Autodesk Inventor part; units mm, degrees
(part 3 of 13)
  arc A798 (17.121, 51.219) -> (17.121, 51.345) centre (17.121, 51.282) ccw
  line L797 (17.121, 51.345) -> (3.5797, 51.345)
  arc A799 (3.5797, 51.345) -> (3.5797, 51.219) centre (3.5797, 51.282) ccw
  line L798 (1.0789, 51.345) -> (1.2725, 51.345)
  arc A800 (1.2725, 51.345) -> (1.2725, 51.471) centre (1.2725, 51.408) ccw
  line L799 (1.2725, 51.471) -> (1.0789, 51.471)
  arc A801 (1.0789, 51.471) -> (1.0789, 51.345) centre (1.0789, 51.408) ccw
  line L800 (2.337, 51.345) -> (2.4628, 51.345)
  arc A802 (2.4628, 51.345) -> (2.4628, 51.471) centre (2.4628, 51.408) ccw
  line L801 (2.4628, 51.471) -> (2.337, 51.471)
  arc A803 (2.337, 51.471) -> (2.337, 51.345) centre (2.337, 51.408) ccw
  line L802 (3.5275, 51.345) -> (17.121, 51.345)
  arc A804 (17.121, 51.345) -> (17.121, 51.471) centre (17.121, 51.408) ccw
  line L803 (17.121, 51.471) -> (3.5275, 51.471)
  arc A805 (3.5275, 51.471) -> (3.5275, 51.345) centre (3.5275, 51.408) ccw
  line L804 (1.0789, 51.471) -> (1.3247, 51.471)
  arc A806 (1.3247, 51.471) -> (1.3247, 51.597) centre (1.3247, 51.534) ccw
  line L805 (1.3247, 51.597) -> (1.0789, 51.597)
  arc A807 (1.0789, 51.597) -> (1.0789, 51.471) centre (1.0789, 51.534) ccw
  line L806 (2.337, 51.471) -> (2.4628, 51.471)
  arc A808 (2.4628, 51.471) -> (2.4628, 51.597) centre (2.4628, 51.534) ccw
  line L807 (2.4628, 51.597) -> (2.337, 51.597)
  arc A809 (2.337, 51.597) -> (2.337, 51.471) centre (2.337, 51.534) ccw
  line L808 (3.4753, 51.471) -> (17.121, 51.471)
  arc A810 (17.121, 51.471) -> (17.121, 51.597) centre (17.121, 51.534) ccw
  line L809 (17.121, 51.597) -> (3.4753, 51.597)
  arc A811 (3.4753, 51.597) -> (3.4753, 51.471) centre (3.4753, 51.534) ccw
  line L810 (1.0789, 51.597) -> (1.389, 51.597)
  arc A812 (1.389, 51.597) -> (1.389, 51.723) centre (1.389, 51.66) ccw
  line L811 (1.389, 51.723) -> (1.0789, 51.723)
  arc A813 (1.0789, 51.723) -> (1.0789, 51.597) centre (1.0789, 51.66) ccw
  line L812 (2.337, 51.597) -> (2.4628, 51.597)
  arc A814 (2.4628, 51.597) -> (2.4628, 51.723) centre (2.4628, 51.66) ccw
  line L813 (2.4628, 51.723) -> (2.337, 51.723)
  arc A815 (2.337, 51.723) -> (2.337, 51.597) centre (2.337, 51.66) ccw
  line L814 (3.4109, 51.597) -> (17.121, 51.597)
  arc A816 (17.121, 51.597) -> (17.121, 51.723) centre (17.121, 51.66) ccw
  line L815 (17.121, 51.723) -> (3.4109, 51.723)
  arc A817 (3.4109, 51.723) -> (3.4109, 51.597) centre (3.4109, 51.66) ccw
  line L816 (1.0789, 51.723) -> (1.515, 51.723)
  arc A818 (1.515, 51.723) -> (1.515, 51.849) centre (1.515, 51.786) ccw
  line L817 (1.515, 51.849) -> (1.0789, 51.849)
  arc A819 (1.0789, 51.849) -> (1.0789, 51.723) centre (1.0789, 51.786) ccw
  line L818 (2.337, 51.723) -> (2.4628, 51.723)
  arc A820 (2.4628, 51.723) -> (2.4628, 51.849) centre (2.4628, 51.786) ccw
  line L819 (2.4628, 51.849) -> (2.337, 51.849)
  arc A821 (2.337, 51.849) -> (2.337, 51.723) centre (2.337, 51.786) ccw
  line L820 (3.2849, 51.723) -> (17.121, 51.723)
  arc A822 (17.121, 51.723) -> (17.121, 51.849) centre (17.121, 51.786) ccw
  line L821 (17.121, 51.849) -> (3.2849, 51.849)
  arc A823 (3.2849, 51.849) -> (3.2849, 51.723) centre (3.2849, 51.786) ccw
  line L822 (1.0789, 51.849) -> (1.641, 51.849)
  arc A824 (1.641, 51.849) -> (1.641, 51.975) centre (1.641, 51.912) ccw
  line L823 (1.641, 51.975) -> (1.0789, 51.975)
  arc A825 (1.0789, 51.975) -> (1.0789, 51.849) centre (1.0789, 51.912) ccw
  line L824 (2.337, 51.849) -> (2.4628, 51.849)
  arc A826 (2.4628, 51.849) -> (2.4628, 51.975) centre (2.4628, 51.912) ccw
  line L825 (2.4628, 51.975) -> (2.337, 51.975)
  arc A827 (2.337, 51.975) -> (2.337, 51.849) centre (2.337, 51.912) ccw
  line L826 (3.1589, 51.849) -> (17.121, 51.849)
  arc A828 (17.121, 51.849) -> (17.121, 51.975) centre (17.121, 51.912) ccw
  line L827 (17.121, 51.975) -> (3.1589, 51.975)
  arc A829 (3.1589, 51.975) -> (3.1589, 51.849) centre (3.1589, 51.912) ccw
  line L828 (1.0789, 51.975) -> (1.8468, 51.975)
  arc A830 (1.8468, 51.975) -> (1.8468, 52.101) centre (1.8468, 52.038) ccw
  line L829 (1.8468, 52.101) -> (1.0789, 52.101)
  arc A831 (1.0789, 52.101) -> (1.0789, 51.975) centre (1.0789, 52.038) ccw
  line L830 (2.337, 51.975) -> (2.4628, 51.975)
  arc A832 (2.4628, 51.975) -> (2.4628, 52.101) centre (2.4628, 52.038) ccw
  line L831 (2.4628, 52.101) -> (2.337, 52.101)
  arc A833 (2.337, 52.101) -> (2.337, 51.975) centre (2.337, 52.038) ccw
  line L832 (2.9532, 51.975) -> (17.121, 51.975)
  arc A834 (17.121, 51.975) -> (17.121, 52.101) centre (17.121, 52.038) ccw
  line L833 (17.121, 52.101) -> (2.9532, 52.101)
  arc A835 (2.9532, 52.101) -> (2.9532, 51.975) centre (2.9532, 52.038) ccw
  line L834 (1.0789, 52.101) -> (2.1509, 52.101)
  arc A836 (2.1509, 52.101) -> (2.1509, 52.227) centre (2.1509, 52.164) ccw
  line L835 (2.1509, 52.227) -> (1.0789, 52.227)
  arc A837 (1.0789, 52.227) -> (1.0789, 52.101) centre (1.0789, 52.164) ccw
  line L836 (2.337, 52.101) -> (2.4628, 52.101)
  arc A838 (2.4628, 52.101) -> (2.4628, 52.227) centre (2.4628, 52.164) ccw
  line L837 (2.4628, 52.227) -> (2.337, 52.227)
  arc A839 (2.337, 52.227) -> (2.337, 52.101) centre (2.337, 52.164) ccw
  line L838 (2.6491, 52.101) -> (17.121, 52.101)
  arc A840 (17.121, 52.101) -> (17.121, 52.227) centre (17.121, 52.164) ccw
  line L839 (17.121, 52.227) -> (2.6491, 52.227)
  arc A841 (2.6491, 52.227) -> (2.6491, 52.101) centre (2.6491, 52.164) ccw
  line L840 (1.0789, 52.227) -> (17.121, 52.227)
  arc A842 (17.121, 52.227) -> (17.121, 52.353) centre (17.121, 52.29) ccw
  line L841 (17.121, 52.353) -> (1.0789, 52.353)
  arc A843 (1.0789, 52.353) -> (1.0789, 52.227) centre (1.0789, 52.29) ccw
  line L842 (1.0789, 52.353) -> (17.121, 52.353)
  arc A844 (17.121, 52.353) -> (17.121, 52.479) centre (17.121, 52.416) ccw
  line L843 (17.121, 52.479) -> (1.0789, 52.479)
  arc A845 (1.0789, 52.479) -> (1.0789, 52.353) centre (1.0789, 52.416) ccw
  line L844 (1.0789, 52.479) -> (17.121, 52.479)
  arc A846 (17.121, 52.479) -> (17.121, 52.605) centre (17.121, 52.542) ccw
  line L845 (17.121, 52.605) -> (1.0789, 52.605)
  arc A847 (1.0789, 52.605) -> (1.0789, 52.479) centre (1.0789, 52.542) ccw
  line L846 (1.0789, 52.605) -> (17.121, 52.605)
  arc A848 (17.121, 52.605) -> (17.121, 52.731) centre (17.121, 52.668) ccw
  line L847 (17.121, 52.731) -> (1.0789, 52.731)
  arc A849 (1.0789, 52.731) -> (1.0789, 52.605) centre (1.0789, 52.668) ccw
  line L848 (1.0789, 52.731) -> (17.121, 52.731)
  arc A850 (17.121, 52.731) -> (17.121, 52.857) centre (17.121, 52.794) ccw
  line L849 (17.121, 52.857) -> (1.0789, 52.857)
  arc A851 (1.0789, 52.857) -> (1.0789, 52.731) centre (1.0789, 52.794) ccw
  line L850 (1.0789, 52.857) -> (17.121, 52.857)
  arc A852 (17.121, 52.857) -> (17.121, 52.983) centre (17.121, 52.92) ccw
  line L851 (17.121, 52.983) -> (1.0789, 52.983)
  arc A853 (1.0789, 52.983) -> (1.0789, 52.857) centre (1.0789, 52.92) ccw
  line L852 (1.0789, 52.983) -> (17.121, 52.983)
  arc A854 (17.121, 52.983) -> (17.121, 53.109) centre (17.121, 53.046) ccw
  line L853 (17.121, 53.109) -> (1.0789, 53.109)
  arc A855 (1.0789, 53.109) -> (1.0789, 52.983) centre (1.0789, 53.046) ccw
  line L854 (1.0789, 53.109) -> (17.121, 53.109)
  arc A856 (17.121, 53.109) -> (17.121, 53.235) centre (17.121, 53.172) ccw
  line L855 (17.121, 53.235) -> (1.0789, 53.235)
  arc A857 (1.0789, 53.235) -> (1.0789, 53.109) centre (1.0789, 53.172) ccw
  line L856 (1.0789, 53.235) -> (17.121, 53.235)
  arc A858 (17.121, 53.235) -> (17.121, 53.361) centre (17.121, 53.298) ccw
  line L857 (17.121, 53.361) -> (1.0789, 53.361)
  arc A859 (1.0789, 53.361) -> (1.0789, 53.235) centre (1.0789, 53.298) ccw
  line L858 (1.0789, 53.361) -> (1.9622, 53.361)
  arc A860 (1.9622, 53.361) -> (1.9622, 53.487) centre (1.9622, 53.424) ccw
  line L859 (1.9622, 53.487) -> (1.0789, 53.487)
  arc A861 (1.0789, 53.487) -> (1.0789, 53.361) centre (1.0789, 53.424) ccw
  line L860 (2.8376, 53.361) -> (17.121, 53.361)
  arc A862 (17.121, 53.361) -> (17.121, 53.487) centre (17.121, 53.424) ccw
  line L861 (17.121, 53.487) -> (2.8376, 53.487)
  arc A863 (2.8376, 53.487) -> (2.8376, 53.361) centre (2.8376, 53.424) ccw
  line L862 (1.0789, 53.487) -> (1.7225, 53.487)
  arc A864 (1.7225, 53.487) -> (1.7225, 53.613) centre (1.7225, 53.55) ccw
  line L863 (1.7225, 53.613) -> (1.0789, 53.613)
  arc A865 (1.0789, 53.613) -> (1.0789, 53.487) centre (1.0789, 53.55) ccw
  line L864 (3.0774, 53.487) -> (17.121, 53.487)
  arc A866 (17.121, 53.487) -> (17.121, 53.613) centre (17.121, 53.55) ccw
  line L865 (17.121, 53.613) -> (3.0774, 53.613)
  arc A867 (3.0774, 53.613) -> (3.0774, 53.487) centre (3.0774, 53.55) ccw
  line L866 (1.0789, 53.613) -> (1.5965, 53.613)
  arc A868 (1.5965, 53.613) -> (1.5965, 53.739) centre (1.5965, 53.676) ccw
  line L867 (1.5965, 53.739) -> (1.0789, 53.739)
  arc A869 (1.0789, 53.739) -> (1.0789, 53.613) centre (1.0789, 53.676) ccw
  line L868 (3.2034, 53.613) -> (7.2516, 53.613)
  arc A870 (7.2516, 53.613) -> (7.2516, 53.739) centre (7.2516, 53.676) ccw
  line L869 (7.2516, 53.739) -> (3.2034, 53.739)
  arc A871 (3.2034, 53.739) -> (3.2034, 53.613) centre (3.2034, 53.676) ccw
  line L870 (8.1482, 53.613) -> (17.121, 53.613)
  arc A872 (17.121, 53.613) -> (17.121, 53.739) centre (17.121, 53.676) ccw
  line L871 (17.121, 53.739) -> (8.1482, 53.739)
  arc A873 (8.1482, 53.739) -> (8.1482, 53.613) centre (8.1482, 53.676) ccw
  line L872 (1.0789, 53.739) -> (1.4705, 53.739)
  arc A874 (1.4705, 53.739) -> (1.4705, 53.865) centre (1.4705, 53.802) ccw
  line L873 (1.4705, 53.865) -> (1.0789, 53.865)
  arc A875 (1.0789, 53.865) -> (1.0789, 53.739) centre (1.0789, 53.802) ccw
  line L874 (3.3294, 53.739) -> (6.9684, 53.739)
  arc A876 (6.9684, 53.739) -> (6.9684, 53.865) centre (6.9684, 53.802) ccw
  line L875 (6.9684, 53.865) -> (3.3294, 53.865)
  arc A877 (3.3294, 53.865) -> (3.3294, 53.739) centre (3.3294, 53.802) ccw
  line L876 (8.4315, 53.739) -> (17.121, 53.739)
  arc A878 (17.121, 53.739) -> (17.121, 53.865) centre (17.121, 53.802) ccw
  line L877 (17.121, 53.865) -> (8.4315, 53.865)
  arc A879 (8.4315, 53.865) -> (8.4315, 53.739) centre (8.4315, 53.802) ccw
  line L878 (1.0789, 53.865) -> (1.4088, 53.865)
  arc A880 (1.4088, 53.865) -> (1.4088, 53.991) centre (1.4088, 53.928) ccw
  line L879 (1.4088, 53.991) -> (1.0789, 53.991)
  arc A881 (1.0789, 53.991) -> (1.0789, 53.865) centre (1.0789, 53.928) ccw
  line L880 (3.391, 53.865) -> (6.8424, 53.865)
  arc A882 (6.8424, 53.865) -> (6.8424, 53.991) centre (6.8424, 53.928) ccw
  line L881 (6.8424, 53.991) -> (3.391, 53.991)
  arc A883 (3.391, 53.991) -> (3.391, 53.865) centre (3.391, 53.928) ccw
  line L882 (8.5575, 53.865) -> (17.121, 53.865)
  arc A884 (17.121, 53.865) -> (17.121, 53.991) centre (17.121, 53.928) ccw
  line L883 (17.121, 53.991) -> (8.5575, 53.991)
  arc A885 (8.5575, 53.991) -> (8.5575, 53.865) centre (8.5575, 53.928) ccw
  line L884 (1.0789, 53.991) -> (1.3567, 53.991)
  arc A886 (1.3567, 53.991) -> (1.3567, 54.117) centre (1.3567, 54.054) ccw
  line L885 (1.3567, 54.117) -> (1.0789, 54.117)
  arc A887 (1.0789, 54.117) -> (1.0789, 53.991) centre (1.0789, 54.054) ccw
  line L886 (3.4431, 53.991) -> (6.7164, 53.991)
  arc A888 (6.7164, 53.991) -> (6.7164, 54.117) centre (6.7164, 54.054) ccw
  line L887 (6.7164, 54.117) -> (3.4431, 54.117)
  arc A889 (3.4431, 54.117) -> (3.4431, 53.991) centre (3.4431, 54.054) ccw
  line L888 (8.6835, 53.991) -> (17.121, 53.991)
  arc A890 (17.121, 53.991) -> (17.121, 54.117) centre (17.121, 54.054) ccw
  line L889 (17.121, 54.117) -> (8.6835, 54.117)
  arc A891 (8.6835, 54.117) -> (8.6835, 53.991) centre (8.6835, 54.054) ccw
  line L890 (1.0789, 54.117) -> (1.3045, 54.117)
  arc A892 (1.3045, 54.117) -> (1.3045, 54.243) centre (1.3045, 54.18) ccw
  line L891 (1.3045, 54.243) -> (1.0789, 54.243)
  arc A893 (1.0789, 54.243) -> (1.0789, 54.117) centre (1.0789, 54.18) ccw
  line L892 (3.4953, 54.117) -> (6.6119, 54.117)
  arc A894 (6.6119, 54.117) -> (6.6119, 54.243) centre (6.6119, 54.18) ccw
  line L893 (6.6119, 54.243) -> (3.4953, 54.243)
  arc A895 (3.4953, 54.243) -> (3.4953, 54.117) centre (3.4953, 54.18) ccw
  line L894 (8.7879, 54.117) -> (17.121, 54.117)
  arc A896 (17.121, 54.117) -> (17.121, 54.243) centre (17.121, 54.18) ccw
  line L895 (17.121, 54.243) -> (8.7879, 54.243)
  arc A897 (8.7879, 54.243) -> (8.7879, 54.117) centre (8.7879, 54.18) ccw
  line L896 (1.0789, 54.243) -> (1.2846, 54.243)
  arc A898 (1.2846, 54.243) -> (1.2846, 54.369) centre (1.2846, 54.306) ccw
  line L897 (1.2846, 54.369) -> (1.0789, 54.369)
  arc A899 (1.0789, 54.369) -> (1.0789, 54.243) centre (1.0789, 54.306) ccw
  line L898 (3.5153, 54.243) -> (6.5597, 54.243)
  arc A900 (6.5597, 54.243) -> (6.5597, 54.369) centre (6.5597, 54.306) ccw
  line L899 (6.5597, 54.369) -> (3.5153, 54.369)
  arc A901 (3.5153, 54.369) -> (3.5153, 54.243) centre (3.5153, 54.306) ccw
  line L900 (8.8401, 54.243) -> (17.121, 54.243)
  arc A902 (17.121, 54.243) -> (17.121, 54.369) centre (17.121, 54.306) ccw
  line L901 (17.121, 54.369) -> (8.8401, 54.369)
  arc A903 (8.8401, 54.369) -> (8.8401, 54.243) centre (8.8401, 54.306) ccw
  line L902 (1.0789, 54.369) -> (1.2846, 54.369)
  arc A904 (1.2846, 54.369) -> (1.2846, 54.495) centre (1.2846, 54.432) ccw
  line L903 (1.2846, 54.495) -> (1.0789, 54.495)
  arc A905 (1.0789, 54.495) -> (1.0789, 54.369) centre (1.0789, 54.432) ccw
  line L904 (3.5153, 54.369) -> (6.5075, 54.369)
  arc A906 (6.5075, 54.369) -> (6.5075, 54.495) centre (6.5075, 54.432) ccw
  line L905 (6.5075, 54.495) -> (3.5153, 54.495)
  arc A907 (3.5153, 54.495) -> (3.5153, 54.369) centre (3.5153, 54.432) ccw
  line L906 (8.8923, 54.369) -> (17.121, 54.369)
  arc A908 (17.121, 54.369) -> (17.121, 54.495) centre (17.121, 54.432) ccw
  line L907 (17.121, 54.495) -> (8.8923, 54.495)
  arc A909 (8.8923, 54.495) -> (8.8923, 54.369) centre (8.8923, 54.432) ccw
  line L908 (1.0789, 54.495) -> (1.2846, 54.495)
  arc A910 (1.2846, 54.495) -> (1.2846, 54.621) centre (1.2846, 54.558) ccw
  line L909 (1.2846, 54.621) -> (1.0789, 54.621)
  arc A911 (1.0789, 54.621) -> (1.0789, 54.495) centre (1.0789, 54.558) ccw
  line L910 (3.5153, 54.495) -> (6.4553, 54.495)
  arc A912 (6.4553, 54.495) -> (6.4553, 54.621) centre (6.4553, 54.558) ccw
  line L911 (6.4553, 54.621) -> (3.5153, 54.621)
  arc A913 (3.5153, 54.621) -> (3.5153, 54.495) centre (3.5153, 54.558) ccw
  line L912 (8.9445, 54.495) -> (17.121, 54.495)
  arc A914 (17.121, 54.495) -> (17.121, 54.621) centre (17.121, 54.558) ccw
  line L913 (17.121, 54.621) -> (8.9445, 54.621)
  arc A915 (8.9445, 54.621) -> (8.9445, 54.495) centre (8.9445, 54.558) ccw
  line L914 (1.0789, 54.621) -> (1.2897, 54.621)
  arc A916 (1.2897, 54.621) -> (1.2897, 54.747) centre (1.2897, 54.684) ccw
  line L915 (1.2897, 54.747) -> (1.0789, 54.747)
  arc A917 (1.0789, 54.747) -> (1.0789, 54.621) centre (1.0789, 54.684) ccw
  line L916 (3.5103, 54.621) -> (6.4346, 54.621)
  arc A918 (6.4346, 54.621) -> (6.4346, 54.747) centre (6.4346, 54.684) ccw
  line L917 (6.4346, 54.747) -> (3.5103, 54.747)
  arc A919 (3.5103, 54.747) -> (3.5103, 54.621) centre (3.5103, 54.684) ccw
  line L918 (8.9653, 54.621) -> (17.121, 54.621)
  arc A920 (17.121, 54.621) -> (17.121, 54.747) centre (17.121, 54.684) ccw
  line L919 (17.121, 54.747) -> (8.9653, 54.747)
  arc A921 (8.9653, 54.747) -> (8.9653, 54.621) centre (8.9653, 54.684) ccw
  line L920 (1.0789, 54.747) -> (1.3419, 54.747)
  arc A922 (1.3419, 54.747) -> (1.3419, 54.873) centre (1.3419, 54.81) ccw
  line L921 (1.3419, 54.873) -> (1.0789, 54.873)
  arc A923 (1.0789, 54.873) -> (1.0789, 54.747) centre (1.0789, 54.81) ccw
  line L922 (3.4581, 54.747) -> (6.4346, 54.747)
  arc A924 (6.4346, 54.747) -> (6.4346, 54.873) centre (6.4346, 54.81) ccw
  line L923 (6.4346, 54.873) -> (3.4581, 54.873)
  arc A925 (3.4581, 54.873) -> (3.4581, 54.747) centre (3.4581, 54.81) ccw
  line L924 (8.9653, 54.747) -> (17.121, 54.747)
  arc A926 (17.121, 54.747) -> (17.121, 54.873) centre (17.121, 54.81) ccw
  line L925 (17.121, 54.873) -> (8.9653, 54.873)
  arc A927 (8.9653, 54.873) -> (8.9653, 54.747) centre (8.9653, 54.81) ccw
  line L926 (1.0789, 54.873) -> (1.3941, 54.873)
  arc A928 (1.3941, 54.873) -> (1.3941, 54.999) centre (1.3941, 54.936) ccw
  line L927 (1.3941, 54.999) -> (1.0789, 54.999)
  arc A929 (1.0789, 54.999) -> (1.0789, 54.873) centre (1.0789, 54.936) ccw
  line L928 (3.4059, 54.873) -> (6.4346, 54.873)
  arc A930 (6.4346, 54.873) -> (6.4346, 54.999) centre (6.4346, 54.936) ccw
  line L929 (6.4346, 54.999) -> (3.4059, 54.999)
  arc A931 (3.4059, 54.999) -> (3.4059, 54.873) centre (3.4059, 54.936) ccw
  line L930 (8.9653, 54.873) -> (17.121, 54.873)
  arc A932 (17.121, 54.873) -> (17.121, 54.999) centre (17.121, 54.936) ccw
  line L931 (17.121, 54.999) -> (8.9653, 54.999)
  arc A933 (8.9653, 54.999) -> (8.9653, 54.873) centre (8.9653, 54.936) ccw
  line L932 (1.0789, 54.999) -> (1.4462, 54.999)
  arc A934 (1.4462, 54.999) -> (1.4462, 55.125) centre (1.4462, 55.062) ccw
  line L933 (1.4462, 55.125) -> (1.0789, 55.125)
  arc A935 (1.0789, 55.125) -> (1.0789, 54.999) centre (1.0789, 55.062) ccw
  line L934 (3.3538, 54.999) -> (6.4346, 54.999)
  arc A936 (6.4346, 54.999) -> (6.4346, 55.125) centre (6.4346, 55.062) ccw
  line L935 (6.4346, 55.125) -> (3.3538, 55.125)
  arc A937 (3.3538, 55.125) -> (3.3538, 54.999) centre (3.3538, 55.062) ccw
  line L936 (8.9653, 54.999) -> (17.121, 54.999)
  arc A938 (17.121, 54.999) -> (17.121, 55.125) centre (17.121, 55.062) ccw
  line L937 (17.121, 55.125) -> (8.9653, 55.125)
  arc A939 (8.9653, 55.125) -> (8.9653, 54.999) centre (8.9653, 55.062) ccw
  line L938 (1.0789, 55.125) -> (1.5606, 55.125)
  arc A940 (1.5606, 55.125) -> (1.5606, 55.251) centre (1.5606, 55.188) ccw
  line L939 (1.5606, 55.251) -> (1.0789, 55.251)
  arc A941 (1.0789, 55.251) -> (1.0789, 55.125) centre (1.0789, 55.188) ccw
  line L940 (3.2393, 55.125) -> (6.4663, 55.125)
  arc A942 (6.4663, 55.125) -> (6.4663, 55.251) centre (6.4663, 55.188) ccw
  line L941 (6.4663, 55.251) -> (3.2393, 55.251)
  arc A943 (3.2393, 55.251) -> (3.2393, 55.125) centre (3.2393, 55.188) ccw
  line L942 (8.9337, 55.125) -> (17.121, 55.125)
  arc A944 (17.121, 55.125) -> (17.121, 55.251) centre (17.121, 55.188) ccw
  line L943 (17.121, 55.251) -> (8.9337, 55.251)
  arc A945 (8.9337, 55.251) -> (8.9337, 55.125) centre (8.9337, 55.188) ccw
  line L944 (1.0789, 55.251) -> (1.6866, 55.251)
  arc A946 (1.6866, 55.251) -> (1.6866, 55.377) centre (1.6866, 55.314) ccw
  line L945 (1.6866, 55.377) -> (1.0789, 55.377)
  arc A947 (1.0789, 55.377) -> (1.0789, 55.251) centre (1.0789, 55.314) ccw
  line L946 (3.1133, 55.251) -> (6.5184, 55.251)
  arc A948 (6.5184, 55.251) -> (6.5184, 55.377) centre (6.5184, 55.314) ccw
  line L947 (6.5184, 55.377) -> (3.1133, 55.377)
  arc A949 (3.1133, 55.377) -> (3.1133, 55.251) centre (3.1133, 55.314) ccw
  line L948 (8.8816, 55.251) -> (17.121, 55.251)
  arc A950 (17.121, 55.251) -> (17.121, 55.377) centre (17.121, 55.314) ccw
  line L949 (17.121, 55.377) -> (8.8816, 55.377)
  arc A951 (8.8816, 55.377) -> (8.8816, 55.251) centre (8.8816, 55.314) ccw
  line L950 (1.0789, 55.377) -> (1.8756, 55.377)
  arc A952 (1.8756, 55.377) -> (1.8756, 55.503) centre (1.8756, 55.44) ccw
  line L951 (1.8756, 55.503) -> (1.0789, 55.503)
  arc A953 (1.0789, 55.503) -> (1.0789, 55.377) centre (1.0789, 55.44) ccw
  line L952 (2.9244, 55.377) -> (6.5706, 55.377)
  arc A954 (6.5706, 55.377) -> (6.5706, 55.503) centre (6.5706, 55.44) ccw
  line L953 (6.5706, 55.503) -> (2.9244, 55.503)
  arc A955 (2.9244, 55.503) -> (2.9244, 55.377) centre (2.9244, 55.44) ccw
  line L954 (8.8294, 55.377) -> (17.121, 55.377)
  arc A956 (17.121, 55.377) -> (17.121, 55.503) centre (17.121, 55.44) ccw
  line L955 (17.121, 55.503) -> (8.8294, 55.503)
  arc A957 (8.8294, 55.503) -> (8.8294, 55.377) centre (8.8294, 55.44) ccw
  line L956 (1.0789, 55.503) -> (6.6228, 55.503)
  arc A958 (6.6228, 55.503) -> (6.6228, 55.629) centre (6.6228, 55.566) ccw
  line L957 (6.6228, 55.629) -> (1.0789, 55.629)
  arc A959 (1.0789, 55.629) -> (1.0789, 55.503) centre (1.0789, 55.566) ccw
  line L958 (8.7772, 55.503) -> (17.121, 55.503)
  arc A960 (17.121, 55.503) -> (17.121, 55.629) centre (17.121, 55.566) ccw
  line L959 (17.121, 55.629) -> (8.7772, 55.629)
  arc A961 (8.7772, 55.629) -> (8.7772, 55.503) centre (8.7772, 55.566) ccw
  line L960 (1.0789, 55.629) -> (6.7425, 55.629)
  arc A962 (6.7425, 55.629) -> (6.7425, 55.755) centre (6.7425, 55.692) ccw
  line L961 (6.7425, 55.755) -> (1.0789, 55.755)
  arc A963 (1.0789, 55.755) -> (1.0789, 55.629) centre (1.0789, 55.692) ccw
  line L962 (8.6574, 55.629) -> (17.121, 55.629)
  arc A964 (17.121, 55.629) -> (17.121, 55.755) centre (17.121, 55.692) ccw
  line L963 (17.121, 55.755) -> (8.6574, 55.755)
  arc A965 (8.6574, 55.755) -> (8.6574, 55.629) centre (8.6574, 55.692) ccw
  line L964 (1.0789, 55.755) -> (6.8685, 55.755)
  arc A966 (6.8685, 55.755) -> (6.8685, 55.881) centre (6.8685, 55.818) ccw
  line L965 (6.8685, 55.881) -> (1.0789, 55.881)
  arc A967 (1.0789, 55.881) -> (1.0789, 55.755) centre (1.0789, 55.818) ccw
  line L966 (8.5314, 55.755) -> (17.121, 55.755)
  arc A968 (17.121, 55.755) -> (17.121, 55.881) centre (17.121, 55.818) ccw
  line L967 (17.121, 55.881) -> (8.5314, 55.881)
  arc A969 (8.5314, 55.881) -> (8.5314, 55.755) centre (8.5314, 55.818) ccw
  line L968 (1.0789, 55.881) -> (7.0105, 55.881)
  arc A970 (7.0105, 55.881) -> (7.0105, 56.007) centre (7.0105, 55.944) ccw
  line L969 (7.0105, 56.007) -> (1.0789, 56.007)
  arc A971 (1.0789, 56.007) -> (1.0789, 55.881) centre (1.0789, 55.944) ccw
  line L970 (8.3895, 55.881) -> (17.121, 55.881)
  arc A972 (17.121, 55.881) -> (17.121, 56.007) centre (17.121, 55.944) ccw
  line L971 (17.121, 56.007) -> (8.3895, 56.007)
  arc A973 (8.3895, 56.007) -> (8.3895, 55.881) centre (8.3895, 55.944) ccw
  line L972 (1.0789, 56.007) -> (7.3147, 56.007)
  arc A974 (7.3147, 56.007) -> (7.3147, 56.133) centre (7.3147, 56.07) ccw
  line L973 (7.3147, 56.133) -> (1.0789, 56.133)
  arc A975 (1.0789, 56.133) -> (1.0789, 56.007) centre (1.0789, 56.07) ccw
  line L974 (8.0853, 56.007) -> (17.121, 56.007)
  arc A976 (17.121, 56.007) -> (17.121, 56.133) centre (17.121, 56.07) ccw
  line L975 (17.121, 56.133) -> (8.0853, 56.133)
  arc A977 (8.0853, 56.133) -> (8.0853, 56.007) centre (8.0853, 56.07) ccw
  line L976 (1.0789, 56.133) -> (17.121, 56.133)
  arc A978 (17.121, 56.133) -> (17.121, 56.259) centre (17.121, 56.196) ccw
  line L977 (17.121, 56.259) -> (1.0789, 56.259)
  arc A979 (1.0789, 56.259) -> (1.0789, 56.133) centre (1.0789, 56.196) ccw
  line L978 (1.0789, 56.259) -> (17.121, 56.259)
  arc A980 (17.121, 56.259) -> (17.121, 56.385) centre (17.121, 56.322) ccw
  line L979 (17.121, 56.385) -> (1.0789, 56.385)
  arc A981 (1.0789, 56.385) -> (1.0789, 56.259) centre (1.0789, 56.322) ccw
  line L980 (1.0789, 56.385) -> (17.121, 56.385)
  arc A982 (17.121, 56.385) -> (17.121, 56.511) centre (17.121, 56.448) ccw
  line L981 (17.121, 56.511) -> (1.0789, 56.511)
  arc A983 (1.0789, 56.511) -> (1.0789, 56.385) centre (1.0789, 56.448) ccw
  line L982 (1.0789, 56.511) -> (17.121, 56.511)
  arc A984 (17.121, 56.511) -> (17.121, 56.637) centre (17.121, 56.574) ccw
  line L983 (17.121, 56.637) -> (1.0789, 56.637)
  arc A985 (1.0789, 56.637) -> (1.0789, 56.511) centre (1.0789, 56.574) ccw
  line L984 (1.0789, 56.637) -> (17.121, 56.637)
  arc A986 (17.121, 56.637) -> (17.121, 56.763) centre (17.121, 56.7) ccw
  line L985 (17.121, 56.763) -> (1.0789, 56.763)
  arc A987 (1.0789, 56.763) -> (1.0789, 56.637) centre (1.0789, 56.7) ccw
  line L986 (1.0789, 56.763) -> (1.9333, 56.763)
  arc A988 (1.9333, 56.763) -> (1.9333, 56.889) centre (1.9333, 56.826) ccw
  line L987 (1.9333, 56.889) -> (1.0789, 56.889)
  arc A989 (1.0789, 56.889) -> (1.0789, 56.763) centre (1.0789, 56.826) ccw
  line L988 (2.337, 56.763) -> (2.4628, 56.763)
  arc A990 (2.4628, 56.763) -> (2.4628, 56.889) centre (2.4628, 56.826) ccw
  line L989 (2.4628, 56.889) -> (2.337, 56.889)
  arc A991 (2.337, 56.889) -> (2.337, 56.763) centre (2.337, 56.826) ccw
  line L990 (2.8665, 56.763) -> (17.121, 56.763)
  arc A992 (17.121, 56.763) -> (17.121, 56.889) centre (17.121, 56.826) ccw
  line L991 (17.121, 56.889) -> (2.8665, 56.889)
  arc A993 (2.8665, 56.889) -> (2.8665, 56.763) centre (2.8665, 56.826) ccw
  line L992 (1.0789, 56.889) -> (1.6769, 56.889)
  arc A994 (1.6769, 56.889) -> (1.6769, 57.015) centre (1.6769, 56.952) ccw
  line L993 (1.6769, 57.015) -> (1.0789, 57.015)
  arc A995 (1.0789, 57.015) -> (1.0789, 56.889) centre (1.0789, 56.952) ccw
  line L994 (2.337, 56.889) -> (2.4628, 56.889)
  arc A996 (2.4628, 56.889) -> (2.4628, 57.015) centre (2.4628, 56.952) ccw
  line L995 (2.4628, 57.015) -> (2.337, 57.015)
  arc A997 (2.337, 57.015) -> (2.337, 56.889) centre (2.337, 56.952) ccw
  line L996 (3.123, 56.889) -> (17.121, 56.889)
  arc A998 (17.121, 56.889) -> (17.121, 57.015) centre (17.121, 56.952) ccw
  line L997 (17.121, 57.015) -> (3.123, 57.015)
  arc A999 (3.123, 57.015) -> (3.123, 56.889) centre (3.123, 56.952) ccw
  line L998 (1.0789, 57.015) -> (1.5509, 57.015)
  arc A1000 (1.5509, 57.015) -> (1.5509, 57.141) centre (1.5509, 57.078) ccw
  line L999 (1.5509, 57.141) -> (1.0789, 57.141)
  arc A1001 (1.0789, 57.141) -> (1.0789, 57.015) centre (1.0789, 57.078) ccw
  line L1000 (2.337, 57.015) -> (2.4628, 57.015)
  arc A1002 (2.4628, 57.015) -> (2.4628, 57.141) centre (2.4628, 57.078) ccw
  line L1001 (2.4628, 57.141) -> (2.337, 57.141)
  arc A1003 (2.337, 57.141) -> (2.337, 57.015) centre (2.337, 57.078) ccw
  line L1002 (3.249, 57.015) -> (17.121, 57.015)
  arc A1004 (17.121, 57.015) -> (17.121, 57.141) centre (17.121, 57.078) ccw
  line L1003 (17.121, 57.141) -> (3.249, 57.141)
  arc A1005 (3.249, 57.141) -> (3.249, 57.015) centre (3.249, 57.078) ccw
  line L1004 (1.0789, 57.141) -> (1.4249, 57.141)
  arc A1006 (1.4249, 57.141) -> (1.4249, 57.267) centre (1.4249, 57.204) ccw
  line L1005 (1.4249, 57.267) -> (1.0789, 57.267)
  arc A1007 (1.0789, 57.267) -> (1.0789, 57.141) centre (1.0789, 57.204) ccw
  line L1006 (2.337, 57.141) -> (2.4628, 57.141)
  arc A1008 (2.4628, 57.141) -> (2.4628, 57.267) centre (2.4628, 57.204) ccw
  line L1007 (2.4628, 57.267) -> (2.337, 57.267)
  arc A1009 (2.337, 57.267) -> (2.337, 57.141) centre (2.337, 57.204) ccw
  line L1008 (3.375, 57.141) -> (17.121, 57.141)
  arc A1010 (17.121, 57.141) -> (17.121, 57.267) centre (17.121, 57.204) ccw
  line L1009 (17.121, 57.267) -> (3.375, 57.267)
  arc A1011 (3.375, 57.267) -> (3.375, 57.141) centre (3.375, 57.204) ccw
  line L1010 (1.0789, 57.267) -> (1.3395, 57.267)
  arc A1012 (1.3395, 57.267) -> (1.3395, 57.393) centre (1.3395, 57.33) ccw
  line L1011 (1.3395, 57.393) -> (1.0789, 57.393)
  arc A1013 (1.0789, 57.393) -> (1.0789, 57.267) centre (1.0789, 57.33) ccw
  line L1012 (2.337, 57.267) -> (2.4628, 57.267)
  arc A1014 (2.4628, 57.267) -> (2.4628, 57.393) centre (2.4628, 57.33) ccw
  line L1013 (2.4628, 57.393) -> (2.337, 57.393)
  arc A1015 (2.337, 57.393) -> (2.337, 57.267) centre (2.337, 57.33) ccw
  line L1014 (3.4603, 57.267) -> (17.121, 57.267)
  arc A1016 (17.121, 57.267) -> (17.121, 57.393) centre (17.121, 57.33) ccw
  line L1015 (17.121, 57.393) -> (3.4603, 57.393)
  arc A1017 (3.4603, 57.393) -> (3.4603, 57.267) centre (3.4603, 57.33) ccw
  line L1016 (1.0789, 57.393) -> (1.2873, 57.393)
  arc A1018 (1.2873, 57.393) -> (1.2873, 57.519) centre (1.2873, 57.456) ccw
  line L1017 (1.2873, 57.519) -> (1.0789, 57.519)
  arc A1019 (1.0789, 57.519) -> (1.0789, 57.393) centre (1.0789, 57.456) ccw
  line L1018 (2.337, 57.393) -> (2.4628, 57.393)
  arc A1020 (2.4628, 57.393) -> (2.4628, 57.519) centre (2.4628, 57.456) ccw
  line L1019 (2.4628, 57.519) -> (2.337, 57.519)
  arc A1021 (2.337, 57.519) -> (2.337, 57.393) centre (2.337, 57.456) ccw
  line L1020 (3.5125, 57.393) -> (17.121, 57.393)
  arc A1022 (17.121, 57.393) -> (17.121, 57.519) centre (17.121, 57.456) ccw
  line L1021 (17.121, 57.519) -> (3.5125, 57.519)
  arc A1023 (3.5125, 57.519) -> (3.5125, 57.393) centre (3.5125, 57.456) ccw
  line L1022 (1.0789, 57.519) -> (1.2351, 57.519)
  arc A1024 (1.2351, 57.519) -> (1.2351, 57.645) centre (1.2351, 57.582) ccw
  line L1023 (1.2351, 57.645) -> (1.0789, 57.645)
  arc A1025 (1.0789, 57.645) -> (1.0789, 57.519) centre (1.0789, 57.582) ccw
  line L1024 (2.337, 57.519) -> (2.4628, 57.519)
  arc A1026 (2.4628, 57.519) -> (2.4628, 57.645) centre (2.4628, 57.582) ccw
  line L1025 (2.4628, 57.645) -> (2.337, 57.645)
  arc A1027 (2.337, 57.645) -> (2.337, 57.519) centre (2.337, 57.582) ccw
  line L1026 (3.5647, 57.519) -> (17.121, 57.519)
  arc A1028 (17.121, 57.519) -> (17.121, 57.645) centre (17.121, 57.582) ccw
  line L1027 (17.121, 57.645) -> (3.5647, 57.645)
  arc A1029 (3.5647, 57.645) -> (3.5647, 57.519) centre (3.5647, 57.582) ccw
  line L1028 (1.0789, 57.645) -> (1.183, 57.645)
  arc A1030 (1.183, 57.645) -> (1.183, 57.771) centre (1.183, 57.708) ccw
  line L1029 (1.183, 57.771) -> (1.0789, 57.771)
  arc A1031 (1.0789, 57.771) -> (1.0789, 57.645) centre (1.0789, 57.708) ccw
  line L1030 (2.337, 57.645) -> (2.4628, 57.645)
  arc A1032 (2.4628, 57.645) -> (2.4628, 57.771) centre (2.4628, 57.708) ccw
  line L1031 (2.4628, 57.771) -> (2.337, 57.771)
  arc A1033 (2.337, 57.771) -> (2.337, 57.645) centre (2.337, 57.708) ccw
  line L1032 (3.6169, 57.645) -> (17.121, 57.645)
  arc A1034 (17.121, 57.645) -> (17.121, 57.771) centre (17.121, 57.708) ccw
  line L1033 (17.121, 57.771) -> (3.6169, 57.771)
  arc A1035 (3.6169, 57.771) -> (3.6169, 57.645) centre (3.6169, 57.708) ccw
  line L1034 (1.0789, 57.771) -> (1.183, 57.771)
  arc A1036 (1.183, 57.771) -> (1.183, 57.897) centre (1.183, 57.834) ccw
  line L1035 (1.183, 57.897) -> (1.0789, 57.897)
  arc A1037 (1.0789, 57.897) -> (1.0789, 57.771) centre (1.0789, 57.834) ccw
  line L1036 (2.337, 57.771) -> (2.4628, 57.771)
  arc A1038 (2.4628, 57.771) -> (2.4628, 57.897) centre (2.4628, 57.834) ccw
  line L1037 (2.4628, 57.897) -> (2.337, 57.897)
  arc A1039 (2.337, 57.897) -> (2.337, 57.771) centre (2.337, 57.834) ccw
  line L1038 (3.6169, 57.771) -> (17.121, 57.771)
  arc A1040 (17.121, 57.771) -> (17.121, 57.897) centre (17.121, 57.834) ccw
  line L1039 (17.121, 57.897) -> (3.6169, 57.897)
  arc A1041 (3.6169, 57.897) -> (3.6169, 57.771) centre (3.6169, 57.834) ccw
  line L1040 (1.0789, 57.897) -> (2.3365, 57.897)
  arc A1042 (2.3365, 57.897) -> (2.3365, 58.023) centre (2.3365, 57.96) ccw
  line L1041 (2.3365, 58.023) -> (1.0789, 58.023)
  arc A1043 (1.0789, 58.023) -> (1.0789, 57.897) centre (1.0789, 57.96) ccw
  line L1042 (2.4634, 57.897) -> (17.121, 57.897)
  arc A1044 (17.121, 57.897) -> (17.121, 58.023) centre (17.121, 57.96) ccw
  line L1043 (17.121, 58.023) -> (2.4634, 58.023)
  arc A1045 (2.4634, 58.023) -> (2.4634, 57.897) centre (2.4634, 57.96) ccw
  line L1044 (1.0789, 58.023) -> (1.183, 58.023)
  arc A1046 (1.183, 58.023) -> (1.183, 58.149) centre (1.183, 58.086) ccw
  line L1045 (1.183, 58.149) -> (1.0789, 58.149)
  arc A1047 (1.0789, 58.149) -> (1.0789, 58.023) centre (1.0789, 58.086) ccw
  line L1046 (2.337, 58.023) -> (2.4628, 58.023)
  arc A1048 (2.4628, 58.023) -> (2.4628, 58.149) centre (2.4628, 58.086) ccw
  line L1047 (2.4628, 58.149) -> (2.337, 58.149)
  arc A1049 (2.337, 58.149) -> (2.337, 58.023) centre (2.337, 58.086) ccw
  line L1048 (3.6169, 58.023) -> (17.121, 58.023)
  arc A1050 (17.121, 58.023) -> (17.121, 58.149) centre (17.121, 58.086) ccw
  line L1049 (17.121, 58.149) -> (3.6169, 58.149)
  arc A1051 (3.6169, 58.149) -> (3.6169, 58.023) centre (3.6169, 58.086) ccw
  line L1050 (1.0789, 58.149) -> (1.1913, 58.149)
  arc A1052 (1.1913, 58.149) -> (1.1913, 58.275) centre (1.1913, 58.212) ccw
  line L1051 (1.1913, 58.275) -> (1.0789, 58.275)
  arc A1053 (1.0789, 58.275) -> (1.0789, 58.149) centre (1.0789, 58.212) ccw
  line L1052 (2.337, 58.149) -> (2.4628, 58.149)
  arc A1054 (2.4628, 58.149) -> (2.4628, 58.275) centre (2.4628, 58.212) ccw
  line L1053 (2.4628, 58.275) -> (2.337, 58.275)
  arc A1055 (2.337, 58.275) -> (2.337, 58.149) centre (2.337, 58.212) ccw
  line L1054 (3.6087, 58.149) -> (17.121, 58.149)
  arc A1056 (17.121, 58.149) -> (17.121, 58.275) centre (17.121, 58.212) ccw
  line L1055 (17.121, 58.275) -> (3.6087, 58.275)
  arc A1057 (3.6087, 58.275) -> (3.6087, 58.149) centre (3.6087, 58.212) ccw
  line L1056 (1.0789, 58.275) -> (1.2435, 58.275)
  arc A1058 (1.2435, 58.275) -> (1.2435, 58.401) centre (1.2435, 58.338) ccw
  line L1057 (1.2435, 58.401) -> (1.0789, 58.401)
  arc A1059 (1.0789, 58.401) -> (1.0789, 58.275) centre (1.0789, 58.338) ccw
  line L1058 (2.337, 58.275) -> (2.4628, 58.275)
  arc A1060 (2.4628, 58.275) -> (2.4628, 58.401) centre (2.4628, 58.338) ccw
  line L1059 (2.4628, 58.401) -> (2.337, 58.401)
  arc A1061 (2.337, 58.401) -> (2.337, 58.275) centre (2.337, 58.338) ccw
  line L1060 (3.5565, 58.275) -> (17.121, 58.275)
  arc A1062 (17.121, 58.275) -> (17.121, 58.401) centre (17.121, 58.338) ccw
  line L1061 (17.121, 58.401) -> (3.5565, 58.401)
  arc A1063 (3.5565, 58.401) -> (3.5565, 58.275) centre (3.5565, 58.338) ccw
  line L1062 (1.0789, 58.401) -> (1.2957, 58.401)
  arc A1064 (1.2957, 58.401) -> (1.2957, 58.527) centre (1.2957, 58.464) ccw
  line L1063 (1.2957, 58.527) -> (1.0789, 58.527)
  arc A1065 (1.0789, 58.527) -> (1.0789, 58.401) centre (1.0789, 58.464) ccw
  line L1064 (2.337, 58.401) -> (2.4628, 58.401)
  arc A1066 (2.4628, 58.401) -> (2.4628, 58.527) centre (2.4628, 58.464) ccw
  line L1065 (2.4628, 58.527) -> (2.337, 58.527)
  arc A1067 (2.337, 58.527) -> (2.337, 58.401) centre (2.337, 58.464) ccw
  line L1066 (3.5043, 58.401) -> (17.121, 58.401)
  arc A1068 (17.121, 58.401) -> (17.121, 58.527) centre (17.121, 58.464) ccw
  line L1067 (17.121, 58.527) -> (3.5043, 58.527)
  arc A1069 (3.5043, 58.527) -> (3.5043, 58.401) centre (3.5043, 58.464) ccw
  line L1068 (1.0789, 58.527) -> (1.3479, 58.527)
  arc A1070 (1.3479, 58.527) -> (1.3479, 58.653) centre (1.3479, 58.59) ccw
  line L1069 (1.3479, 58.653) -> (1.0789, 58.653)
  arc A1071 (1.0789, 58.653) -> (1.0789, 58.527) centre (1.0789, 58.59) ccw
  line L1070 (2.337, 58.527) -> (2.4628, 58.527)
  arc A1072 (2.4628, 58.527) -> (2.4628, 58.653) centre (2.4628, 58.59) ccw
  line L1071 (2.4628, 58.653) -> (2.337, 58.653)
  arc A1073 (2.337, 58.653) -> (2.337, 58.527) centre (2.337, 58.59) ccw
  line L1072 (3.4521, 58.527) -> (7.3869, 58.527)
  arc A1074 (7.3869, 58.527) -> (7.3869, 58.653) centre (7.3869, 58.59) ccw
  line L1073 (7.3869, 58.653) -> (3.4521, 58.653)
  arc A1075 (3.4521, 58.653) -> (3.4521, 58.527) centre (3.4521, 58.59) ccw
  line L1074 (7.637, 58.527) -> (7.7628, 58.527)
  arc A1076 (7.7628, 58.527) -> (7.7628, 58.653) centre (7.7628, 58.59) ccw
  line L1075 (7.7628, 58.653) -> (7.637, 58.653)
  arc A1077 (7.637, 58.653) -> (7.637, 58.527) centre (7.637, 58.59) ccw
  line L1076 (8.0129, 58.527) -> (17.121, 58.527)
  arc A1078 (17.121, 58.527) -> (17.121, 58.653) centre (17.121, 58.59) ccw
  line L1077 (17.121, 58.653) -> (8.0129, 58.653)
  arc A1079 (8.0129, 58.653) -> (8.0129, 58.527) centre (8.0129, 58.59) ccw
  line L1078 (1.0789, 58.653) -> (1.445, 58.653)
  arc A1080 (1.445, 58.653) -> (1.445, 58.779) centre (1.445, 58.716) ccw
  line L1079 (1.445, 58.779) -> (1.0789, 58.779)
  arc A1081 (1.0789, 58.779) -> (1.0789, 58.653) centre (1.0789, 58.716) ccw
  line L1080 (2.337, 58.653) -> (2.4628, 58.653)
  arc A1082 (2.4628, 58.653) -> (2.4628, 58.779) centre (2.4628, 58.716) ccw
  line L1081 (2.4628, 58.779) -> (2.337, 58.779)
  arc A1083 (2.337, 58.779) -> (2.337, 58.653) centre (2.337, 58.716) ccw
  line L1082 (3.3549, 58.653) -> (7.0827, 58.653)
  arc A1084 (7.0827, 58.653) -> (7.0827, 58.779) centre (7.0827, 58.716) ccw
  line L1083 (7.0827, 58.779) -> (3.3549, 58.779)
  arc A1085 (3.3549, 58.779) -> (3.3549, 58.653) centre (3.3549, 58.716) ccw
  line L1084 (7.637, 58.653) -> (7.7628, 58.653)
  arc A1086 (7.7628, 58.653) -> (7.7628, 58.779) centre (7.7628, 58.716) ccw
  line L1085 (7.7628, 58.779) -> (7.637, 58.779)
  arc A1087 (7.637, 58.779) -> (7.637, 58.653) centre (7.637, 58.716) ccw
  line L1086 (8.3171, 58.653) -> (17.121, 58.653)
  arc A1088 (17.121, 58.653) -> (17.121, 58.779) centre (17.121, 58.716) ccw
  line L1087 (17.121, 58.779) -> (8.3171, 58.779)
  arc A1089 (8.3171, 58.779) -> (8.3171, 58.653) centre (8.3171, 58.716) ccw
  line L1088 (1.0789, 58.779) -> (1.571, 58.779)
  arc A1090 (1.571, 58.779) -> (1.571, 58.905) centre (1.571, 58.842) ccw
  line L1089 (1.571, 58.905) -> (1.0789, 58.905)
  arc A1091 (1.0789, 58.905) -> (1.0789, 58.779) centre (1.0789, 58.842) ccw
  line L1090 (2.337, 58.779) -> (2.4628, 58.779)
  arc A1092 (2.4628, 58.779) -> (2.4628, 58.905) centre (2.4628, 58.842) ccw
  line L1091 (2.4628, 58.905) -> (2.337, 58.905)
  arc A1093 (2.337, 58.905) -> (2.337, 58.779) centre (2.337, 58.842) ccw
  line L1092 (3.2289, 58.779) -> (6.8647, 58.779)
  arc A1094 (6.8647, 58.779) -> (6.8647, 58.905) centre (6.8647, 58.842) ccw
  line L1093 (6.8647, 58.905) -> (3.2289, 58.905)
  arc A1095 (3.2289, 58.905) -> (3.2289, 58.779) centre (3.2289, 58.842) ccw
  line L1094 (7.637, 58.779) -> (7.7628, 58.779)
  arc A1096 (7.7628, 58.779) -> (7.7628, 58.905) centre (7.7628, 58.842) ccw
  line L1095 (7.7628, 58.905) -> (7.637, 58.905)
  arc A1097 (7.637, 58.905) -> (7.637, 58.779) centre (7.637, 58.842) ccw
  line L1096 (8.5352, 58.779) -> (17.121, 58.779)
  arc A1098 (17.121, 58.779) -> (17.121, 58.905) centre (17.121, 58.842) ccw
  line L1097 (17.121, 58.905) -> (8.5352, 58.905)
  arc A1099 (8.5352, 58.905) -> (8.5352, 58.779) centre (8.5352, 58.842) ccw
  line L1098 (1.0789, 58.905) -> (1.697, 58.905)
  arc A1100 (1.697, 58.905) -> (1.697, 59.031) centre (1.697, 58.968) ccw
  line L1099 (1.697, 59.031) -> (1.0789, 59.031)
  arc A1101 (1.0789, 59.031) -> (1.0789, 58.905) centre (1.0789, 58.968) ccw
  line L1100 (2.337, 58.905) -> (2.4628, 58.905)
  arc A1102 (2.4628, 58.905) -> (2.4628, 59.031) centre (2.4628, 58.968) ccw
  line L1101 (2.4628, 59.031) -> (2.337, 59.031)
  arc A1103 (2.337, 59.031) -> (2.337, 58.905) centre (2.337, 58.968) ccw
  line L1102 (3.1029, 58.905) -> (6.7387, 58.905)
  arc A1104 (6.7387, 58.905) -> (6.7387, 59.031) centre (6.7387, 58.968) ccw
  line L1103 (6.7387, 59.031) -> (3.1029, 59.031)
  arc A1105 (3.1029, 59.031) -> (3.1029, 58.905) centre (3.1029, 58.968) ccw
  line L1104 (7.637, 58.905) -> (7.7628, 58.905)
  arc A1106 (7.7628, 58.905) -> (7.7628, 59.031) centre (7.7628, 58.968) ccw
  line L1105 (7.7628, 59.031) -> (7.637, 59.031)
  arc A1107 (7.637, 59.031) -> (7.637, 58.905) centre (7.637, 58.968) ccw
  line L1106 (8.6612, 58.905) -> (17.121, 58.905)
  arc A1108 (17.121, 58.905) -> (17.121, 59.031) centre (17.121, 58.968) ccw
  line L1107 (17.121, 59.031) -> (8.6612, 59.031)
  arc A1109 (8.6612, 59.031) -> (8.6612, 58.905) centre (8.6612, 58.968) ccw
  line L1108 (1.0789, 59.031) -> (1.9819, 59.031)
  arc A1110 (1.9819, 59.031) -> (1.9819, 59.157) centre (1.9819, 59.094) ccw
  line L1109 (1.9819, 59.157) -> (1.0789, 59.157)
  arc A1111 (1.0789, 59.157) -> (1.0789, 59.031) centre (1.0789, 59.094) ccw
  line L1110 (2.337, 59.031) -> (2.4628, 59.031)
  arc A1112 (2.4628, 59.031) -> (2.4628, 59.157) centre (2.4628, 59.094) ccw
  line L1111 (2.4628, 59.157) -> (2.337, 59.157)
  arc A1113 (2.337, 59.157) -> (2.337, 59.031) centre (2.337, 59.094) ccw
  line L1112 (2.8181, 59.031) -> (6.6127, 59.031)
  arc A1114 (6.6127, 59.031) -> (6.6127, 59.157) centre (6.6127, 59.094) ccw
  line L1113 (6.6127, 59.157) -> (2.8181, 59.157)
  arc A1115 (2.8181, 59.157) -> (2.8181, 59.031) centre (2.8181, 59.094) ccw
  line L1114 (7.637, 59.031) -> (7.7628, 59.031)
  arc A1116 (7.7628, 59.031) -> (7.7628, 59.157) centre (7.7628, 59.094) ccw
  line L1115 (7.7628, 59.157) -> (7.637, 59.157)
  arc A1117 (7.637, 59.157) -> (7.637, 59.031) centre (7.637, 59.094) ccw
  line L1116 (8.7872, 59.031) -> (17.121, 59.031)
  arc A1118 (17.121, 59.031) -> (17.121, 59.157) centre (17.121, 59.094) ccw
  line L1117 (17.121, 59.157) -> (8.7872, 59.157)
  arc A1119 (8.7872, 59.157) -> (8.7872, 59.031) centre (8.7872, 59.094) ccw
  line L1118 (1.0789, 59.157) -> (6.5185, 59.157)
  arc A1120 (6.5185, 59.157) -> (6.5185, 59.283) centre (6.5185, 59.22) ccw
  line L1119 (6.5185, 59.283) -> (1.0789, 59.283)
  arc A1121 (1.0789, 59.283) -> (1.0789, 59.157) centre (1.0789, 59.22) ccw
  line L1120 (7.637, 59.157) -> (7.7628, 59.157)
  arc A1122 (7.7628, 59.157) -> (7.7628, 59.283) centre (7.7628, 59.22) ccw
  line L1121 (7.7628, 59.283) -> (7.637, 59.283)
  arc A1123 (7.637, 59.283) -> (7.637, 59.157) centre (7.637, 59.22) ccw
  line L1122 (8.8813, 59.157) -> (17.121, 59.157)
  arc A1124 (17.121, 59.157) -> (17.121, 59.283) centre (17.121, 59.22) ccw
  line L1123 (17.121, 59.283) -> (8.8813, 59.283)
  arc A1125 (8.8813, 59.283) -> (8.8813, 59.157) centre (8.8813, 59.22) ccw
  line L1124 (1.0789, 59.283) -> (6.4663, 59.283)
  arc A1126 (6.4663, 59.283) -> (6.4663, 59.409) centre (6.4663, 59.346) ccw
  line L1125 (6.4663, 59.409) -> (1.0789, 59.409)
  arc A1127 (1.0789, 59.409) -> (1.0789, 59.283) centre (1.0789, 59.346) ccw
  line L1126 (7.637, 59.283) -> (7.7628, 59.283)
  arc A1128 (7.7628, 59.283) -> (7.7628, 59.409) centre (7.7628, 59.346) ccw
  line L1127 (7.7628, 59.409) -> (7.637, 59.409)
  arc A1129 (7.637, 59.409) -> (7.637, 59.283) centre (7.637, 59.346) ccw
  line L1128 (8.9335, 59.283) -> (17.121, 59.283)
  arc A1130 (17.121, 59.283) -> (17.121, 59.409) centre (17.121, 59.346) ccw
  line L1129 (17.121, 59.409) -> (8.9335, 59.409)
  arc A1131 (8.9335, 59.409) -> (8.9335, 59.283) centre (8.9335, 59.346) ccw
  line L1130 (1.0789, 59.409) -> (6.4141, 59.409)
  arc A1132 (6.4141, 59.409) -> (6.4141, 59.535) centre (6.4141, 59.472) ccw
  line L1131 (6.4141, 59.535) -> (1.0789, 59.535)
  arc A1133 (1.0789, 59.535) -> (1.0789, 59.409) centre (1.0789, 59.472) ccw
  line L1132 (7.637, 59.409) -> (7.7628, 59.409)
  arc A1134 (7.7628, 59.409) -> (7.7628, 59.535) centre (7.7628, 59.472) ccw
  line L1133 (7.7628, 59.535) -> (7.637, 59.535)
  arc A1135 (7.637, 59.535) -> (7.637, 59.409) centre (7.637, 59.472) ccw
  line L1134 (8.9857, 59.409) -> (17.121, 59.409)
  arc A1136 (17.121, 59.409) -> (17.121, 59.535) centre (17.121, 59.472) ccw
  line L1135 (17.121, 59.535) -> (8.9857, 59.535)
  arc A1137 (8.9857, 59.535) -> (8.9857, 59.409) centre (8.9857, 59.472) ccw
  line L1136 (1.0789, 59.535) -> (6.3619, 59.535)
  arc A1138 (6.3619, 59.535) -> (6.3619, 59.661) centre (6.3619, 59.598) ccw
  line L1137 (6.3619, 59.661) -> (1.0789, 59.661)
  arc A1139 (1.0789, 59.661) -> (1.0789, 59.535) centre (1.0789, 59.598) ccw
  line L1138 (7.637, 59.535) -> (7.7628, 59.535)
  arc A1140 (7.7628, 59.535) -> (7.7628, 59.661) centre (7.7628, 59.598) ccw
  line L1139 (7.7628, 59.661) -> (7.637, 59.661)
  arc A1141 (7.637, 59.661) -> (7.637, 59.535) centre (7.637, 59.598) ccw
  line L1140 (9.0379, 59.535) -> (17.121, 59.535)
  arc A1142 (17.121, 59.535) -> (17.121, 59.661) centre (17.121, 59.598) ccw
  line L1141 (17.121, 59.661) -> (9.0379, 59.661)
  arc A1143 (9.0379, 59.661) -> (9.0379, 59.535) centre (9.0379, 59.598) ccw
  line L1142 (1.0789, 59.661) -> (6.333, 59.661)
  arc A1144 (6.333, 59.661) -> (6.333, 59.787) centre (6.333, 59.724) ccw
  line L1143 (6.333, 59.787) -> (1.0789, 59.787)
  arc A1145 (1.0789, 59.787) -> (1.0789, 59.661) centre (1.0789, 59.724) ccw
  line L1144 (7.637, 59.661) -> (7.7628, 59.661)
  arc A1146 (7.7628, 59.661) -> (7.7628, 59.787) centre (7.7628, 59.724) ccw
  line L1145 (7.7628, 59.787) -> (7.637, 59.787)
  arc A1147 (7.637, 59.787) -> (7.637, 59.661) centre (7.637, 59.724) ccw
  line L1146 (9.0669, 59.661) -> (17.121, 59.661)
  arc A1148 (17.121, 59.661) -> (17.121, 59.787) centre (17.121, 59.724) ccw
  line L1147 (17.121, 59.787) -> (9.0669, 59.787)
  arc A1149 (9.0669, 59.787) -> (9.0669, 59.661) centre (9.0669, 59.724) ccw
  line L1148 (1.0789, 59.787) -> (6.333, 59.787)
  arc A1150 (6.333, 59.787) -> (6.333, 59.913) centre (6.333, 59.85) ccw
  line L1149 (6.333, 59.913) -> (1.0789, 59.913)
  arc A1151 (1.0789, 59.913) -> (1.0789, 59.787) centre (1.0789, 59.85) ccw
  line L1150 (7.637, 59.787) -> (7.7628, 59.787)
  arc A1152 (7.7628, 59.787) -> (7.7628, 59.913) centre (7.7628, 59.85) ccw
  line L1151 (7.7628, 59.913) -> (7.637, 59.913)
  arc A1153 (7.637, 59.913) -> (7.637, 59.787) centre (7.637, 59.85) ccw
  line L1152 (9.0669, 59.787) -> (17.121, 59.787)
  arc A1154 (17.121, 59.787) -> (17.121, 59.913) centre (17.121, 59.85) ccw
  line L1153 (17.121, 59.913) -> (9.0669, 59.913)
  arc A1155 (9.0669, 59.913) -> (9.0669, 59.787) centre (9.0669, 59.85) ccw
  line L1154 (1.0789, 59.913) -> (7.6365, 59.913)
  arc A1156 (7.6365, 59.913) -> (7.6365, 60.039) centre (7.6365, 59.976) ccw
  line L1155 (7.6365, 60.039) -> (1.0789, 60.039)
  arc A1157 (1.0789, 60.039) -> (1.0789, 59.913) centre (1.0789, 59.976) ccw
  line L1156 (7.7634, 59.913) -> (17.121, 59.913)
  arc A1158 (17.121, 59.913) -> (17.121, 60.039) centre (17.121, 59.976) ccw
  line L1157 (17.121, 60.039) -> (7.7634, 60.039)
  arc A1159 (7.7634, 60.039) -> (7.7634, 59.913) centre (7.7634, 59.976) ccw
  line L1158 (1.0789, 60.039) -> (6.333, 60.039)
  arc A1160 (6.333, 60.039) -> (6.333, 60.165) centre (6.333, 60.102) ccw
  line L1159 (6.333, 60.165) -> (1.0789, 60.165)
  arc A1161 (1.0789, 60.165) -> (1.0789, 60.039) centre (1.0789, 60.102) ccw
  line L1160 (7.637, 60.039) -> (7.7628, 60.039)
  arc A1162 (7.7628, 60.039) -> (7.7628, 60.165) centre (7.7628, 60.102) ccw
  line L1161 (7.7628, 60.165) -> (7.637, 60.165)
  arc A1163 (7.637, 60.165) -> (7.637, 60.039) centre (7.637, 60.102) ccw
  line L1162 (9.0669, 60.039) -> (17.121, 60.039)
  arc A1164 (17.121, 60.039) -> (17.121, 60.165) centre (17.121, 60.102) ccw
  line L1163 (17.121, 60.165) -> (9.0669, 60.165)
  arc A1165 (9.0669, 60.165) -> (9.0669, 60.039) centre (9.0669, 60.102) ccw
  line L1164 (1.0789, 60.165) -> (6.3397, 60.165)
  arc A1166 (6.3397, 60.165) -> (6.3397, 60.291) centre (6.3397, 60.228) ccw
  line L1165 (6.3397, 60.291) -> (1.0789, 60.291)
  arc A1167 (1.0789, 60.291) -> (1.0789, 60.165) centre (1.0789, 60.228) ccw
  line L1166 (7.637, 60.165) -> (7.7628, 60.165)
  arc A1168 (7.7628, 60.165) -> (7.7628, 60.291) centre (7.7628, 60.228) ccw
  line L1167 (7.7628, 60.291) -> (7.637, 60.291)
  arc A1169 (7.637, 60.291) -> (7.637, 60.165) centre (7.637, 60.228) ccw
  line L1168 (9.0603, 60.165) -> (17.121, 60.165)
  arc A1170 (17.121, 60.165) -> (17.121, 60.291) centre (17.121, 60.228) ccw
  line L1169 (17.121, 60.291) -> (9.0603, 60.291)
  arc A1171 (9.0603, 60.291) -> (9.0603, 60.165) centre (9.0603, 60.228) ccw
  line L1170 (1.0789, 60.291) -> (6.3919, 60.291)
  arc A1172 (6.3919, 60.291) -> (6.3919, 60.417) centre (6.3919, 60.354) ccw
  line L1171 (6.3919, 60.417) -> (1.0789, 60.417)
  arc A1173 (1.0789, 60.417) -> (1.0789, 60.291) centre (1.0789, 60.354) ccw
  line L1172 (7.637, 60.291) -> (7.7628, 60.291)
  arc A1174 (7.7628, 60.291) -> (7.7628, 60.417) centre (7.7628, 60.354) ccw
  line L1173 (7.7628, 60.417) -> (7.637, 60.417)
  arc A1175 (7.637, 60.417) -> (7.637, 60.291) centre (7.637, 60.354) ccw
  line L1174 (9.0081, 60.291) -> (17.121, 60.291)
  arc A1176 (17.121, 60.291) -> (17.121, 60.417) centre (17.121, 60.354) ccw
  line L1175 (17.121, 60.417) -> (9.0081, 60.417)
  arc A1177 (9.0081, 60.417) -> (9.0081, 60.291) centre (9.0081, 60.354) ccw
  line L1176 (1.0789, 60.417) -> (6.4441, 60.417)
  arc A1178 (6.4441, 60.417) -> (6.4441, 60.543) centre (6.4441, 60.48) ccw
  line L1177 (6.4441, 60.543) -> (1.0789, 60.543)
  arc A1179 (1.0789, 60.543) -> (1.0789, 60.417) centre (1.0789, 60.48) ccw
  line L1178 (7.637, 60.417) -> (7.7628, 60.417)
  arc A1180 (7.7628, 60.417) -> (7.7628, 60.543) centre (7.7628, 60.48) ccw
  line L1179 (7.7628, 60.543) -> (7.637, 60.543)
  arc A1181 (7.637, 60.543) -> (7.637, 60.417) centre (7.637, 60.48) ccw
  line L1180 (8.9559, 60.417) -> (17.121, 60.417)
  arc A1182 (17.121, 60.417) -> (17.121, 60.543) centre (17.121, 60.48) ccw
  line L1181 (17.121, 60.543) -> (8.9559, 60.543)
  arc A1183 (8.9559, 60.543) -> (8.9559, 60.417) centre (8.9559, 60.48) ccw
  line L1182 (1.0789, 60.543) -> (6.4963, 60.543)
  arc A1184 (6.4963, 60.543) -> (6.4963, 60.669) centre (6.4963, 60.606) ccw
  line L1183 (6.4963, 60.669) -> (1.0789, 60.669)
  arc A1185 (1.0789, 60.669) -> (1.0789, 60.543) centre (1.0789, 60.606) ccw
  line L1184 (7.637, 60.543) -> (7.7628, 60.543)
  arc A1186 (7.7628, 60.543) -> (7.7628, 60.669) centre (7.7628, 60.606) ccw
  line L1185 (7.7628, 60.669) -> (7.637, 60.669)
  arc A1187 (7.637, 60.669) -> (7.637, 60.543) centre (7.637, 60.606) ccw
  line L1186 (8.9037, 60.543) -> (17.121, 60.543)
  arc A1188 (17.121, 60.543) -> (17.121, 60.669) centre (17.121, 60.606) ccw
  line L1187 (17.121, 60.669) -> (8.9037, 60.669)
  arc A1189 (8.9037, 60.669) -> (8.9037, 60.543) centre (8.9037, 60.606) ccw
  line L1188 (1.0789, 60.669) -> (6.5588, 60.669)
  arc A1190 (6.5588, 60.669) -> (6.5588, 60.795) centre (6.5588, 60.732) ccw
  line L1189 (6.5588, 60.795) -> (1.0789, 60.795)
  arc A1191 (1.0789, 60.795) -> (1.0789, 60.669) centre (1.0789, 60.732) ccw
  line L1190 (7.637, 60.669) -> (7.7628, 60.669)
  arc A1192 (7.7628, 60.669) -> (7.7628, 60.795) centre (7.7628, 60.732) ccw
  line L1191 (7.7628, 60.795) -> (7.637, 60.795)
  arc A1193 (7.637, 60.795) -> (7.637, 60.669) centre (7.637, 60.732) ccw
  line L1192 (8.8411, 60.669) -> (17.121, 60.669)
  arc A1194 (17.121, 60.669) -> (17.121, 60.795) centre (17.121, 60.732) ccw
  line L1193 (17.121, 60.795) -> (8.8411, 60.795)
  arc A1195 (8.8411, 60.795) -> (8.8411, 60.669) centre (8.8411, 60.732) ccw
  line L1194 (1.0789, 60.795) -> (6.6848, 60.795)
  arc A1196 (6.6848, 60.795) -> (6.6848, 60.921) centre (6.6848, 60.858) ccw
  line L1195 (6.6848, 60.921) -> (1.0789, 60.921)